Autodesk Inventor part; units mm, degrees
(part 2 of 3)
sketch "Sketch41" plane through (0, 15, 0) normal (0, 1, 0) x (1, 0, 0)
  line L0 (-15.5, 102.8) -> (-15.5, 122.8) projected
  line L1 (-15.5, 112.8) -> (-5.5, 112.8)
  line L2 (-5.5, 102.8) -> (-5.5, 122.8) projected
  line L3 (-5.5, 72.8) -> (-5.5, 92.8) projected
  line L4 (-5.5, 82.8) -> (-15.5, 82.8)
  line L5 (-15.5, 72.8) -> (-15.5, 92.8) projected
  line L6 (-35.5, 72.8) -> (-35.5, 92.8) projected
  line L7 (-35.5, 82.8) -> (-45.5, 82.8)
  line L8 (-45.5, 72.8) -> (-45.5, 92.8) projected
  line L9 (-65.5, 72.8) -> (-65.5, 92.8) projected
  line L10 (-65.5, 82.8) -> (-75.5, 82.8)
  line L11 (-75.5, 72.8) -> (-75.5, 92.8) projected
  line L12 (-75.5, 62.8) -> (-75.5, 42.8) projected
  line L13 (-75.5, 52.8) -> (-65.5, 52.8)
  line L14 (-65.5, 42.8) -> (-65.5, 62.8) projected
  line L15 (-45.5, 42.8) -> (-45.5, 62.8) projected
  line L16 (-45.5, 52.8) -> (-35.5, 52.8)
  line L17 (-35.5, 42.8) -> (-35.5, 62.8) projected
  line L18 (-15.5, 52.8) -> (-5.5, 52.8)
  line L19 (-5.5, 42.8) -> (-5.5, 62.8) projected
  line L20 (-5.5, 32.8) -> (-5.5, 12.8) projected
  line L21 (-5.5, 22.8) -> (-15.5, 22.8)
  line L22 (-15.5, 32.8) -> (-15.5, 12.8) projected
  line L23 (-45.5, 22.8) -> (-35.5, 22.8)
  line L24 (-35.5, 32.8) -> (-35.5, 12.8) projected
  line L25 (-65.5, 22.8) -> (-75.5, 22.8)
  line L26 (-75.5, 32.8) -> (-75.5, 12.8) projected
  line L27 (-70.5, 82.8) -> (-70.5, 93.8)
  line L28 (-70.5, 82.8) -> (-59.5, 82.8) construction
  line L29 (-70.5, 93.8) -> (-70.5, 71.8)
  line L30 (-40.5, 82.8) -> (-40.5, 93.8)
  line L31 (-40.5, 93.8) -> (-40.5, 71.8)
  line L32 (-10.5, 82.8) -> (-10.5, 93.8)
  line L33 (-10.5, 93.8) -> (-10.5, 71.8)
  line L34 (-10.5, 52.8) -> (-10.5, 63.8)
  line L35 (-10.5, 63.8) -> (-10.5, 41.8)
  line L36 (-40.5, 52.8) -> (-40.5, 63.8)
  line L37 (-40.5, 63.8) -> (-40.5, 41.8)
  line L38 (-70.5, 52.8) -> (-70.5, 63.8)
  line L39 (-70.5, 63.8) -> (-70.5, 41.8)
  line L40 (-70.5, 22.8) -> (-70.5, 33.8)
  line L41 (-70.5, 33.8) -> (-70.5, 11.8)
  line L42 (-40.5, 22.8) -> (-40.5, 33.8)
  line L43 (-45.5, 32.8) -> (-35.5, 32.8) projected
  line L44 (-40.5, 22.8) -> (-29.5, 22.8) construction
  line L45 (-40.5, 33.8) -> (-40.5, 11.8)
  line L46 (-10.5, 22.8) -> (-10.5, 33.8)
  line L47 (-10.5, 33.8) -> (-10.5, 11.8)
  line L48 (-10.5, 112.8) -> (-10.5, 123.8)
  line L49 (-10.5, 123.8) -> (-10.5, 101.8)
  line L50 (-10.5, 101.8) -> (0.5, 112.8)
  line L51 (0.5, 112.8) -> (-10.5, 123.8)
  line L52 (-21.5, 112.8) -> (-10.5, 101.8)
  line L53 (-10.5, 123.8) -> (-21.5, 112.8)
  line L54 (-70.5, 93.8) -> (-59.5, 82.8)
  line L55 (-70.5, 71.8) -> (-59.5, 82.8)
  line L56 (-70.5, 71.8) -> (-81.5, 82.8)
  line L57 (-81.5, 82.8) -> (-70.5, 93.8)
  line L58 (-40.5, 93.8) -> (-29.5, 82.8)
  line L59 (-29.5, 82.8) -> (-40.5, 71.8)
  line L60 (-51.5, 82.8) -> (-40.5, 71.8)
  line L61 (-51.5, 82.8) -> (-40.5, 93.8)
  line L62 (-10.5, 93.8) -> (0.5, 82.8)
  line L63 (0.5, 82.8) -> (-10.5, 71.8)
  line L64 (-21.5, 82.8) -> (-10.5, 93.8)
  line L65 (-21.5, 82.8) -> (-10.5, 71.8)
  line L66 (-10.5, 63.8) -> (0.5, 52.8)
  line L67 (-10.5, 63.8) -> (5.0563, 63.8) construction
  line L68 (0.5, 52.8) -> (-10.5, 41.8)
  line L69 (-10.5, 41.8) -> (-21.5, 52.8)
  line L70 (-21.5, 52.8) -> (-10.5, 63.8)
  line L71 (-40.5, 63.8) -> (-29.5, 52.8)
  line L72 (-29.5, 52.8) -> (-40.5, 41.8)
  line L73 (-51.5, 52.8) -> (-40.5, 63.8)
  line L74 (-51.5, 52.8) -> (-40.5, 41.8)
  line L75 (-70.5, 63.8) -> (-59.5, 52.8)
  line L76 (-59.5, 52.8) -> (-70.5, 41.8)
  line L77 (-81.5, 52.8) -> (-70.5, 41.8)
  line L78 (-81.5, 52.8) -> (-70.5, 63.8)
  line L79 (-70.5, 33.8) -> (-59.5, 22.8)
  line L80 (-59.5, 22.8) -> (-70.5, 11.8)
  line L81 (-81.5, 22.8) -> (-70.5, 11.8)
  line L82 (-81.5, 22.8) -> (-70.5, 33.8)
  line L83 (-40.5, 33.8) -> (-29.5, 22.8)
  line L84 (-40.5, 11.8) -> (-29.5, 22.8)
  line L85 (-40.5, 11.8) -> (-51.5, 22.8)
  line L86 (-51.5, 22.8) -> (-40.5, 33.8)
  line L87 (-10.5, 33.8) -> (0.5, 22.8)
  line L88 (0.5, 22.8) -> (-10.5, 11.8)
  line L89 (-21.5, 22.8) -> (-10.5, 11.8)
  line L90 (-21.5, 22.8) -> (-10.5, 33.8)
  line L91 (-5.5, 102.8) -> (-15.5, 102.8) projected
  line L92 (-15.5, 122.8) -> (-5.5, 122.8)
  line L93 (-5.5, 122.8) -> (-5.5, 102.8)
  line L94 (-5.5, 102.8) -> (-15.5, 102.8)
  line L95 (-15.5, 102.8) -> (-15.5, 122.8)
  line L96 (-15.5, 92.8) -> (-5.5, 92.8) projected
  line L97 (-15.5, 92.8) -> (-5, 92.8)
  line L98 (-5, 92.8) -> (-5, 72.8)
  line L99 (-5, 72.8) -> (-15.5, 72.8)
  line L100 (-15.5, 72.8) -> (-15.5, 92.8)
  line L101 (-45.5, 92.8) -> (-35.5, 92.8)
  line L102 (-35.5, 92.8) -> (-35.5, 72.8)
  line L103 (-35.5, 72.8) -> (-45.5, 72.8)
  line L104 (-45.5, 72.8) -> (-45.5, 92.8)
  line L105 (-75.5, 92.8) -> (-65, 92.8)
  line L106 (-65, 92.8) -> (-65, 72.8)
  line L107 (-65, 72.8) -> (-75.5, 72.8)
  line L108 (-75.5, 72.8) -> (-75.5, 92.8)
  line L109 (-75.5, 62.8) -> (-65.5, 62.8) projected
  line L110 (-75.5, 62.8) -> (-65.5, 62.8)
  line L111 (-65.5, 62.8) -> (-65.5, 42.8)
  line L112 (-65.5, 42.8) -> (-75.5, 42.8)
  line L113 (-75.5, 42.8) -> (-75.5, 62.8)
  line L114 (-45.5, 62.8) -> (-35.5, 62.8) projected
  line L115 (-45.5, 62.8) -> (-35.5, 62.8)
  line L116 (-35.5, 62.8) -> (-35.5, 42.8)
  line L117 (-35.5, 42.8) -> (-45.5, 42.8)
  line L118 (-45.5, 42.8) -> (-45.5, 62.8)
  line L119 (-15.5, 62.8) -> (-5.5, 62.8) projected
  line L120 (-5.5, 42.8) -> (-15.5, 42.8) projected
  line L121 (-15.5, 62.8) -> (-5.5, 62.8)
  line L122 (-5.5, 62.8) -> (-5.5, 42.8)
  line L123 (-5.5, 42.8) -> (-15.5, 42.8)
  line L124 (-15.5, 42.8) -> (-15.5, 62.8)
  line L125 (-15.5, 32.8) -> (-5.5, 32.8)
  line L126 (-5.5, 32.8) -> (-5.5, 12.8)
  line L127 (-5.5, 12.8) -> (-15.5, 12.8)
  line L128 (-15.5, 12.8) -> (-15.5, 32.8)
  line L129 (-45.5, 32.8) -> (-45.5, 12.8) projected
  line L130 (-45.5, 32.8) -> (-35.5, 32.8)
  line L131 (-35.5, 32.8) -> (-35.5, 12.8)
  line L132 (-35.5, 12.8) -> (-45.5, 12.8)
  line L133 (-45.5, 12.8) -> (-45.5, 32.8)
  line L134 (-75.5, 32.8) -> (-65.5, 32.8)
  line L135 (-65.5, 32.8) -> (-65.5, 12.8)
  line L136 (-65.5, 12.8) -> (-75.5, 12.8)
  line L137 (-75.5, 12.8) -> (-75.5, 32.8)
  point P0 (0, 0)
  point P1 (-41.5, 42.8)
  point P2 (-45.5, 46.8)
  point P3 (-39.5, 42.8)
  point P4 (-35.5, 46.8)
  point P5 (-39.5, 62.8)
  point P6 (-35.5, 58.8)
  point P7 (-41.5, 62.8)
  point P8 (-45.5, 58.8)
  point P9 (-41.5, 12.8)
  point P10 (-45.5, 16.8)
  point P11 (-39.5, 12.8)
  point P12 (-35.5, 16.8)
  point P13 (-39.5, 32.8)
  point P14 (-35.5, 28.8)
  point P15 (-45.5, 28.8)
  point P16 (-41.5, 32.8)
  point P17 (-71.5, 12.8)
  point P18 (-75.5, 16.8)
  point P19 (-69.5, 12.8)
  point P20 (-65.5, 16.8)
  point P21 (-65.5, 28.8)
  point P22 (-69.5, 32.8)
  point P23 (-71.5, 32.8)
  point P24 (-75.5, 28.8)
  point P25 (-71.5, 42.8)
  point P26 (-75.5, 46.8)
  point P27 (-69.5, 42.8)
  point P28 (-65.5, 46.8)
  point P29 (-69.5, 62.8)
  point P30 (-65.5, 58.8)
  point P31 (-71.5, 62.8)
  point P32 (-75.5, 58.8)
  point P33 (-71.5, 72.8)
  point P34 (-75.5, 76.8)
  point P35 (-69.5, 72.8)
  point P36 (-65.5, 76.8)
  point P37 (-71.5, 92.8)
  point P38 (-75.5, 88.8)
  point P39 (-69.5, 92.8)
  point P40 (-65.5, 88.8)
  point P41 (-39.5, 72.8)
  point P42 (-35.5, 76.8)
  point P43 (-41.5, 72.8)
  point P44 (-45.5, 76.8)
  point P45 (-39.5, 92.8)
  point P46 (-35.5, 88.8)
  point P47 (-41.5, 92.8)
  point P48 (-45.5, 88.8)
  point P49 (-11.5, 12.8)
  point P50 (-15.5, 16.8)
  point P51 (-9.5, 12.8)
  point P52 (-5.5, 16.8)
  point P53 (-9.5, 32.8)
  point P54 (-5.5, 28.8)
  point P55 (-11.5, 32.8)
  point P56 (-15.5, 28.8)
  point P57 (-9.5, 62.8)
  point P58 (-5.5, 58.8)
  point P59 (-15.5, 58.8)
  point P60 (-11.5, 62.8)
  point P61 (-15.5, 46.8)
  point P62 (-11.5, 42.8)
  point P63 (-9.5, 42.8)
  point P64 (-5.5, 46.8)
  point P65 (-9.5, 72.8)
  point P66 (-5.5, 76.8)
  point P67 (-9.5, 92.8)
  point P68 (-5.5, 88.8)
  point P69 (-11.5, 92.8)
  point P70 (-15.5, 88.8)
  point P71 (-11.5, 72.8)
  point P72 (-15.5, 76.8)
  point P73 (-11.5, 102.8)
  point P74 (-15.5, 106.8)
  point P75 (-9.5, 102.8)
  point P76 (-5.5, 106.8)
  point P77 (-9.5, 122.8)
  point P78 (-5.5, 118.8)
  point P79 (-11.5, 122.8)
  point P80 (-15.5, 118.8)
  dimension "d189" = 11
  dimension "d190" = 90
  dimension "d191" = 22
  dimension "d192" = 11
  dimension "d193" = 22
  dimension "d194" = 11
  dimension "d195" = 22
  dimension "d196" = 11
  dimension "d197" = 22
  dimension "d198" = 11
  dimension "d199" = 22
  dimension "d200" = 11
  dimension "d201" = 22
  dimension "d202" = 11
  dimension "d203" = 22
  dimension "d204" = 11
  dimension "d205" = 90
  dimension "d206" = 22
  dimension "d207" = 11
  dimension "d208" = 22
  dimension "d209" = 11
  dimension "d210" = 22
  dimension "d211" = 45
  dimension "d212" = 45
  constraints: 226 end point, 36 perpendicular, 27 midpoint, 23 point on line, 22 parallel, 13 horizontal, 9 vertical, 3 equal length
  measures "d189" distance of L27.start L27.end
  measures "d190" angle of L28 L27
  measures "d191" distance of L27.end L29.end
  measures "d192" distance of L30.start L30.end
  measures "d193" distance of L30.end L31.end
  measures "d194" distance of L32.start L32.end
  measures "d195" distance of L32.end L33.end
  measures "d196" distance of L34.start L34.end
  measures "d197" distance of L34.end L35.end
  measures "d198" distance of L36.start L36.end
  measures "d199" distance of L36.end L37.end
  measures "d200" distance of L38.start L38.end
  measures "d201" distance of L38.end L39.end
  measures "d202" distance of L40.start L40.end
  measures "d203" distance of L40.end L41.end
  measures "d204" distance of L42.start L42.end
  measures "d205" angle of L44 L42
  measures "d206" distance of L42.end L45.end
  measures "d207" distance of L46.start L46.end
  measures "d208" distance of L46.end L47.end
  measures "d209" distance of L48.start L48.end
  measures "d210" distance of L48.end L49.end
  measures "d211" angle of L50 L49
  measures "d212" angle of L66 L67
extrude "Extrusion39" add sketch "Sketch41" along normal blind 3 contours L0 L52 L91 | L0 L92 L53 | L50 L2 L91 | L51 L92 L2 | L99 L63 L3 | L62 L96 L3 | L99 L5 L65 | L5 L96 L64 | L103 L59 L6 | L58 L101 L6 | L103 L8 L60 | L8 L101 L61 | L107 L55 L9 | L54 L105 L9 | L107 L11 L56 | L11 L105 L57 | L109 L78 L12 | L77 L112 L12 | L109 L14 L75 | L14 L112 L76 | L15 L74 L117 | L15 L114 L73 | L72 L17 L117 | L71 L114 L17 | L69 L120 L124 | L124 L119 L70 | L19 L120 L68 | L66 L119 L19 | L20 L87 L125 | L20 L127 L88 | L90 L22 L125 | L89 L127 L22 | L129 L43 L86 | L85 L132 L129 | L83 L43 L24 | L24 L132 L84 | L79 L134 L135 | L135 L136 L80 | L26 L134 L82 | L81 L136 L26
chamfer "Chamfer9" distance 2.5 distance2 3 1 edges at (-73.5, 18, -90.8) measured on face at (-73.8536, 18, -91.1536)
chamfer "Chamfer10" distance 2.5 distance2 3 1 edges at (-67.5, 18, -90.8) measured on face at (-67.1464, 18, -91.1536)
chamfer "Chamfer11" distance 2.5 distance2 3 1 edges at (-67.5, 18, -74.8) measured on face at (-67.1464, 18, -74.4464)
chamfer "Chamfer12" distance 2.5 distance2 3 1 edges at (-73.5, 18, -74.8) measured on face at (-73.8536, 18, -74.4464)
chamfer "Chamfer13" distance 2.5 distance2 3 1 edges at (-73.5, 18, -60.8) measured on face at (-73.8536, 18, -61.1536)
chamfer "Chamfer14" distance 2.5 distance2 3 1 edges at (-67.5, 18, -60.8) measured on face at (-67.1464, 18, -61.1536)
chamfer "Chamfer15" distance 2.5 distance2 3 1 edges at (-67.5, 18, -44.8) measured on face at (-67.1464, 18, -44.4464)
chamfer "Chamfer16" distance 2.5 distance2 3 1 edges at (-73.5, 18, -44.8) measured on face at (-73.8536, 18, -44.4464)
chamfer "Chamfer17" distance 2.5 distance2 3 1 edges at (-73.5, 18, -30.8) measured on face at (-73.8536, 18, -31.1536)
chamfer "Chamfer18" distance 2.5 distance2 3 1 edges at (-67.5, 18, -30.8) measured on face at (-67.1464, 18, -31.1536)
chamfer "Chamfer19" distance 2.5 distance2 3 1 edges at (-67.5, 18, -14.8) measured on face at (-67.1464, 18, -14.4464)
chamfer "Chamfer20" distance 2.5 distance2 3 1 edges at (-73.5, 18, -14.8) measured on face at (-73.8536, 18, -14.4464)
chamfer "Chamfer21" distance 2.5 distance2 3 1 edges at (-43.5, 18, -30.8) measured on face at (-43.8536, 18, -31.1536)
chamfer "Chamfer22" distance 2.5 distance2 3 1 edges at (-43.5, 18, -14.8) measured on face at (-43.8536, 18, -14.4464)
chamfer "Chamfer23" distance 2.5 distance2 3 1 edges at (-37.5, 18, -14.8) measured on face at (-37.1464, 18, -14.4464)
chamfer "Chamfer24" distance 2.5 distance2 3 1 edges at (-37.5, 18, -30.8) measured on face at (-37.1464, 18, -31.1536)
chamfer "Chamfer25" distance 2.5 distance2 3 1 edges at (-43.5, 18, -60.8) measured on face at (-43.8536, 18, -61.1536)
chamfer "Chamfer26" distance 2.5 distance2 3 1 edges at (-43.5, 18, -44.8) measured on face at (-43.8536, 18, -44.4464)
chamfer "Chamfer27" distance 2.5 distance2 3 1 edges at (-37.5, 18, -44.8) measured on face at (-37.1464, 18, -44.4464)
chamfer "Chamfer28" distance 2.5 distance2 3 1 edges at (-37.5, 18, -60.8) measured on face at (-37.1464, 18, -61.1536)
chamfer "Chamfer29" distance 2.5 distance2 3 1 edges at (-13.5, 18, -30.8) measured on face at (-13.8536, 18, -31.1536)
chamfer "Chamfer30" distance 2.5 distance2 3 1 edges at (-13.5, 18, -14.8) measured on face at (-13.8536, 18, -14.4464)
chamfer "Chamfer31" distance 2.5 distance2 3 1 edges at (-7.5, 18, -14.8) measured on face at (-7.1464, 18, -14.4464)
chamfer "Chamfer32" distance 2.5 distance2 3 1 edges at (-7.5, 18, -30.8) measured on face at (-7.1464, 18, -31.1536)
chamfer "Chamfer33" distance 2.5 distance2 3 1 edges at (-13.5, 18, -60.8) measured on face at (-13.8536, 18, -61.1536)
chamfer "Chamfer34" distance 2.5 distance2 3 1 edges at (-13.5, 18, -44.8) measured on face at (-13.8536, 18, -44.4464)
chamfer "Chamfer35" distance 2.5 distance2 3 1 edges at (-7.5, 18, -44.8) measured on face at (-7.1464, 18, -44.4464)
chamfer "Chamfer36" distance 2.5 distance2 3 1 edges at (-7.5, 18, -60.8) measured on face at (-7.1464, 18, -61.1536)
chamfer "Chamfer37" distance 2.5 distance2 3 1 edges at (-13.5, 18, -90.8) measured on face at (-13.8536, 18, -91.1536)
chamfer "Chamfer38" distance 2.5 distance2 3 1 edges at (-13.5, 18, -74.8) measured on face at (-13.8536, 18, -74.4464)
chamfer "Chamfer39" distance 2.5 distance2 3 1 edges at (-7.5, 18, -74.8) measured on face at (-7.1464, 18, -74.4464)
chamfer "Chamfer40" distance 2.5 distance2 3 1 edges at (-7.5, 18, -90.8) measured on face at (-7.1464, 18, -91.1536)
chamfer "Chamfer41" distance 2.5 distance2 3 1 edges at (-13.5, 18, -120.8) measured on face at (-13.8536, 18, -121.1536)
chamfer "Chamfer42" distance 2.5 distance2 3 1 edges at (-7.5, 18, -120.8) measured on face at (-7.1464, 18, -121.1536)
chamfer "Chamfer43" distance 2.5 distance2 3 1 edges at (-7.5, 18, -104.8) measured on face at (-7.1464, 18, -104.4464)
chamfer "Chamfer44" distance 2.5 distance2 3 1 edges at (-13.5, 18, -104.8) measured on face at (-13.8536, 18, -104.4464)
chamfer "Chamfer45" distance 2.5 distance2 3 1 edges at (-43.5, 18, -90.8) measured on face at (-43.8536, 18, -91.1536)
chamfer "Chamfer46" distance 2.5 distance2 3 1 edges at (-43.5, 18, -74.8) measured on face at (-43.8536, 18, -74.4464)
chamfer "Chamfer47" distance 2.5 distance2 3 1 edges at (-37.5, 18, -90.8) measured on face at (-37.1464, 18, -91.1536)
chamfer "Chamfer48" distance 2.5 distance2 3 1 edges at (-37.5, 18, -74.8) measured on face at (-37.1464, 18, -74.4464)
sketch "Sketch42" plane through (0, 15, 0) normal (0, 1, 0) x (1, 0, 0)
  line L0 (-69.5, 102.8) -> (-65.5, 106.8) projected
  line L1 (-65.5, 106.8) -> (-65.5, 118.8) projected
  line L2 (-65.5, 118.8) -> (-69.5, 122.8) projected
  line L3 (-71.5, 122.8) -> (-69.5, 122.8) projected
  line L4 (-71.5, 122.8) -> (-75.5, 118.8) projected
  line L5 (-75.5, 118.8) -> (-75.5, 106.8) projected
  line L6 (-75.5, 106.8) -> (-71.5, 102.8) projected
  line L7 (-69.5, 102.8) -> (-71.5, 102.8) projected
  line L8 (-39.5, 102.8) -> (-35.5, 106.8) projected
  line L9 (-35.5, 106.8) -> (-35.5, 118.8) projected
  line L10 (-35.5, 118.8) -> (-39.5, 122.8) projected
  line L11 (-41.5, 122.8) -> (-39.5, 122.8) projected
  line L12 (-41.5, 122.8) -> (-45.5, 118.8) projected
  line L13 (-45.5, 118.8) -> (-45.5, 106.8) projected
  line L14 (-45.5, 106.8) -> (-41.5, 102.8) projected
  line L15 (-39.5, 102.8) -> (-41.5, 102.8) projected
  line L16 (-9.5, 102.8) -> (-5.5, 106.8) projected
  line L17 (-5.5, 106.8) -> (-5.5, 118.8) projected
  line L18 (-5.5, 118.8) -> (-9.5, 122.8) projected
  line L19 (-11.5, 122.8) -> (-9.5, 122.8) projected
  line L20 (-11.5, 122.8) -> (-15.5, 118.8) projected
  line L21 (-15.5, 118.8) -> (-15.5, 106.8) projected
  line L22 (-15.5, 106.8) -> (-11.5, 102.8) projected
  line L23 (-9.5, 102.8) -> (-11.5, 102.8) projected
  line L24 (-5.5, 88.8) -> (-9.5, 92.8) projected
  line L25 (-11.5, 92.8) -> (-9.5, 92.8) projected
  line L26 (-11.5, 92.8) -> (-15.5, 88.8) projected
  line L27 (-15.5, 88.8) -> (-15.5, 76.8) projected
  line L28 (-15.5, 76.8) -> (-11.5, 72.8) projected
  line L29 (-9.5, 72.8) -> (-11.5, 72.8) projected
  line L30 (-9.5, 72.8) -> (-5.5, 76.8) projected
  line L31 (-5.5, 76.8) -> (-5.5, 88.8) projected
  line L32 (-45.5, 76.8) -> (-41.5, 72.8) projected
  line L33 (-39.5, 72.8) -> (-41.5, 72.8) projected
  line L34 (-39.5, 72.8) -> (-35.5, 76.8) projected
  line L35 (-35.5, 76.8) -> (-35.5, 88.8) projected
  line L36 (-35.5, 88.8) -> (-39.5, 92.8) projected
  line L37 (-41.5, 92.8) -> (-39.5, 92.8) projected
  line L38 (-41.5, 92.8) -> (-45.5, 88.8) projected
  line L39 (-45.5, 88.8) -> (-45.5, 76.8) projected
  line L40 (-69.5, 72.8) -> (-65.5, 76.8) projected
  line L41 (-65.5, 76.8) -> (-65.5, 88.8) projected
  line L42 (-65.5, 88.8) -> (-69.5, 92.8) projected
  line L43 (-71.5, 92.8) -> (-69.5, 92.8) projected
  line L44 (-71.5, 92.8) -> (-75.5, 88.8) projected
  line L45 (-75.5, 88.8) -> (-75.5, 76.8) projected
  line L46 (-75.5, 76.8) -> (-71.5, 72.8) projected
  line L47 (-69.5, 72.8) -> (-71.5, 72.8) projected
  line L48 (-75.5, 58.8) -> (-75.5, 46.8) projected
  line L49 (-69.5, 42.8) -> (-65.5, 46.8) projected
  line L50 (-65.5, 46.8) -> (-65.5, 58.8) projected
  line L51 (-65.5, 58.8) -> (-69.5, 62.8) projected
  line L52 (-71.5, 62.8) -> (-69.5, 62.8) projected
  line L53 (-71.5, 62.8) -> (-75.5, 58.8) projected
  line L54 (-75.5, 58.8) -> (-75.5, 46.8) projected
  line L55 (-75.5, 46.8) -> (-71.5, 42.8) projected
  line L56 (-69.5, 42.8) -> (-71.5, 42.8) projected
  line L57 (-39.5, 42.8) -> (-35.5, 46.8) projected
  line L58 (-35.5, 46.8) -> (-35.5, 58.8) projected
  line L59 (-35.5, 58.8) -> (-39.5, 62.8) projected
  line L60 (-41.5, 62.8) -> (-39.5, 62.8) projected
  line L61 (-41.5, 62.8) -> (-45.5, 58.8) projected
  line L62 (-45.5, 58.8) -> (-45.5, 46.8) projected
  line L63 (-45.5, 46.8) -> (-41.5, 42.8) projected
  line L64 (-39.5, 42.8) -> (-41.5, 42.8) projected
  line L65 (-11.5, 62.8) -> (-15.5, 58.8) projected
  line L66 (-15.5, 58.8) -> (-15.5, 46.8) projected
  line L67 (-15.5, 46.8) -> (-11.5, 42.8) projected
  line L68 (-9.5, 42.8) -> (-11.5, 42.8) projected
  line L69 (-9.5, 42.8) -> (-5.5, 46.8) projected
  line L70 (-5.5, 46.8) -> (-5.5, 58.8) projected
  line L71 (-5.5, 58.8) -> (-9.5, 62.8) projected
  line L72 (-11.5, 62.8) -> (-9.5, 62.8) projected
  line L73 (-9.5, 12.8) -> (-5.5, 16.8) projected
  line L74 (-5.5, 16.8) -> (-5.5, 28.8) projected
  line L75 (-5.5, 28.8) -> (-9.5, 32.8) projected
  line L76 (-11.5, 32.8) -> (-9.5, 32.8) projected
  line L77 (-11.5, 32.8) -> (-15.5, 28.8) projected
  line L78 (-15.5, 28.8) -> (-15.5, 16.8) projected
  line L79 (-15.5, 16.8) -> (-11.5, 12.8) projected
  line L80 (-9.5, 12.8) -> (-11.5, 12.8) projected
  line L81 (-39.5, 12.8) -> (-35.5, 16.8) projected
  line L82 (-35.5, 16.8) -> (-35.5, 28.8) projected
  line L83 (-35.5, 28.8) -> (-39.5, 32.8) projected
  line L84 (-41.5, 32.8) -> (-39.5, 32.8) projected
  line L85 (-41.5, 32.8) -> (-45.5, 28.8) projected
  line L86 (-45.5, 28.8) -> (-45.5, 16.8) projected
  line L87 (-45.5, 16.8) -> (-41.5, 12.8) projected
  line L88 (-39.5, 12.8) -> (-41.5, 12.8) projected
  line L89 (-69.5, 12.8) -> (-65.5, 16.8) projected
  line L90 (-65.5, 16.8) -> (-65.5, 28.8) projected
  line L91 (-65.5, 28.8) -> (-69.5, 32.8) projected
  line L92 (-71.5, 32.8) -> (-69.5, 32.8) projected
  line L93 (-71.5, 32.8) -> (-75.5, 28.8) projected
  line L94 (-75.5, 28.8) -> (-75.5, 16.8) projected
  line L95 (-75.5, 16.8) -> (-71.5, 12.8) projected
  line L96 (-69.5, 12.8) -> (-71.5, 12.8) projected
  point P0 (0, 0)
extrude "Extrusion40" cut sketch "Sketch42" against normal blind 3
sketch "Sketch43" plane through (0, 12, 0) normal (0, 1, 0) x (1, 0, 0)
  line L0 (-91.1439, 136.9955) -> (37.6505, 136.9955)
  line L1 (37.6505, 136.9955) -> (37.6505, 0)
  line L2 (37.6505, 0) -> (-91.1439, 0)
  line L3 (-91.1439, 0) -> (-91.1439, 136.9955)
  point P0 (0, 0)
  constraints: 8 end point, 2 parallel, 1 horizontal, 1 perpendicular
extrude "Extrusion41" cut sketch "Sketch43" along normal blind 10
sketch "Sketch44" plane through (0, 12, 0) normal (0, 1, 0) x (1, 0, 0)
  line L0 (-75.5, 102.8) -> (-75.5, 122.8) projected
  line L1 (-65.5, 12.8) -> (-75.5, 12.8) projected
  line L2 (-75.5, 122.8) -> (-74.5, 122.8)
  line L3 (-74.5, 122.8) -> (-74.5, 12.8)
  line L4 (-74.5, 12.8) -> (-75.5, 12.8)
  line L5 (-75.5, 12.8) -> (-75.5, 122.8)
  line L6 (-65.5, 122.8) -> (-65.5, 102.8) projected
  line L7 (-65.5, 122.8) -> (-66.5, 122.8)
  line L8 (-66.5, 122.8) -> (-66.5, 12.8)
  line L9 (-66.5, 12.8) -> (-65.5, 12.8)
  line L10 (-65.5, 12.8) -> (-65.5, 122.8)
  line L11 (-35.5, 12.8) -> (-45.5, 12.8) projected
  line L12 (-45.5, 12.8) -> (-44.5, 12.8)
  line L13 (-44.5, 12.8) -> (-44.5, 122.8)
  line L14 (-44.5, 122.8) -> (-45.5, 122.8)
  line L15 (-45.5, 122.8) -> (-45.5, 12.8)
  line L16 (-35.5, 122.8) -> (-36.5, 122.8)
  line L17 (-36.5, 122.8) -> (-36.5, 12.8)
  line L18 (-36.5, 12.8) -> (-35.5, 12.8)
  line L19 (-35.5, 12.8) -> (-35.5, 122.8)
  line L20 (-15.5, 122.8) -> (-5.5, 122.8) projected
  line L21 (-5.5, 12.8) -> (-15.5, 12.8) projected
  line L22 (-15.5, 122.8) -> (-14.5, 122.8)
  line L23 (-14.5, 122.8) -> (-14.5, 12.8)
  line L24 (-14.5, 12.8) -> (-15.5, 12.8)
  line L25 (-15.5, 12.8) -> (-15.5, 122.8)
  line L26 (-5.5, 122.8) -> (-6.5, 122.8)
  line L27 (-6.5, 122.8) -> (-6.5, 12.8)
  line L28 (-6.5, 12.8) -> (-5.5, 12.8)
  line L29 (-5.5, 12.8) -> (-5.5, 122.8)
  point P0 (0, 0)
  dimension "d339" = 1
  dimension "d340" = 1
  dimension "d341" = 1
  dimension "d342" = 1
  dimension "d343" = 1
  dimension "d344" = 1
  constraints: 48 end point, 12 parallel, 7 point on line, 6 horizontal, 6 perpendicular
  measures "d339" distance of L3.end L4.end
  measures "d340" distance of L9.end L8.end
  measures "d341" distance of L14.end L13.end
  measures "d342" distance of L18.end L17.end
  measures "d343" distance of L23.end L24.end
  measures "d344" distance of L28.end L27.end
extrude "Extrusion42" cut sketch "Sketch44" against normal blind 7 contours L0 L2 L3 L1 L5 | L1 L8 L7 L6 L10 | L11 L17 L16 L19 | L11 L15 L14 L13 | L20 L23 L21 L25 | L20 L29 L21 L27
sketch "Sketch45" plane through (0, 12, 0) normal (0, 1, 0) x (1, 0, 0)
  line L0 (-74.5, 122.8) -> (-74.5, 102.8) projected
  line L1 (-74.5, 122.8) -> (-66.5, 122.8)
  line L2 (-66.5, 122.8) -> (-66.5, 125.8)
  line L3 (-66.5, 125.8) -> (-74.5, 125.8)
  line L4 (-74.5, 125.8) -> (-74.5, 122.8)
  line L5 (-66.5, 102.8) -> (-66.5, 122.8) projected
  line L6 (-66.5, 102.8) -> (-74.5, 102.8)
  line L7 (-74.5, 102.8) -> (-74.5, 99.8)
  line L8 (-74.5, 99.8) -> (-66.5, 99.8)
  line L9 (-66.5, 99.8) -> (-66.5, 102.8)
  line L10 (-74.5, 92.8) -> (-66.5, 92.8) projected
  line L11 (-74.5, 92.8) -> (-66.5, 92.8)
  line L12 (-66.5, 92.8) -> (-66.5, 95.8)
  line L13 (-66.5, 95.8) -> (-74.5, 95.8)
  line L14 (-74.5, 95.8) -> (-74.5, 92.8)
  line L15 (-66.5, 72.8) -> (-74.5, 72.8) projected
  line L16 (-74.5, 72.8) -> (-66.5, 72.8)
  line L17 (-66.5, 72.8) -> (-66.5, 69.8)
  line L18 (-66.5, 69.8) -> (-74.5, 69.8)
  line L19 (-74.5, 69.8) -> (-74.5, 72.8)
  line L20 (-74.5, 62.8) -> (-66.5, 62.8)
  line L21 (-66.5, 62.8) -> (-66.5, 65.8)
  line L22 (-66.5, 65.8) -> (-74.5, 65.8)
  line L23 (-74.5, 65.8) -> (-74.5, 62.8)
  line L24 (-66.5, 42.8) -> (-74.5, 42.8) projected
  line L25 (-74.5, 42.8) -> (-66.5, 42.8)
  line L26 (-66.5, 42.8) -> (-66.5, 39.8)
  line L27 (-66.5, 39.8) -> (-74.5, 39.8)
  line L28 (-74.5, 39.8) -> (-74.5, 42.8)
  line L29 (-74.5, 32.8) -> (-66.5, 32.8) projected
  line L30 (-74.5, 32.8) -> (-66.5, 32.8)
  line L31 (-66.5, 32.8) -> (-66.5, 35.8)
  line L32 (-66.5, 35.8) -> (-74.5, 35.8)
  line L33 (-74.5, 35.8) -> (-74.5, 32.8)
  line L34 (-66.5, 12.8) -> (-74.5, 12.8) projected
  line L35 (-74.5, 12.8) -> (-66.5, 12.8)
  line L36 (-66.5, 12.8) -> (-66.5, 9.8)
  line L37 (-66.5, 9.8) -> (-74.5, 9.8)
  line L38 (-74.5, 9.8) -> (-74.5, 12.8)
  point P0 (0, 0)
  dimension "d347" = 3
  dimension "d348" = 3
  dimension "d349" = 8
  dimension "d350" = 3
  dimension "d351" = 3
  dimension "d352" = 8
  dimension "d353" = 3
  dimension "d354" = 8
  dimension "d355" = 3
  dimension "d356" = 8
  dimension "d357" = 3
  dimension "d358" = 8
  dimension "d359" = 3
  constraints: 64 end point, 16 parallel, 8 horizontal, 8 perpendicular, 2 point on line
  measures "d347" distance of L2.end L1.end
  measures "d348" distance of L7.end L6.end
  measures "d349" distance of L13.end L12.end
  measures "d350" distance of L12.end L11.end
  measures "d351" distance of L16.end L17.end
  measures "d352" distance of L22.end L21.end
  measures "d353" distance of L21.end L20.end
  measures "d354" distance of L26.end L27.end
  measures "d355" distance of L25.end L26.end
  measures "d356" distance of L32.end L31.end
  measures "d357" distance of L31.end L30.end
  measures "d358" distance of L36.end L37.end
  measures "d359" distance of L35.end L36.end
extrude "Extrusion43" add sketch "Sketch45" against normal blind 7 contours L4 L3 L2 L1 | L6 L9 L8 L7 | L14 L13 L12 L10 | L17 L18 L19 L15 | L23 L22 L21 L20 | L26 L27 L28 L24 | L33 L32 L31 L29 | L36 L37 L38 L34
sketch "Sketch46" plane through (0, 12, 0) normal (0, 1, 0) x (1, 0, 0)
  line L0 (-74.5, 99.8) -> (-74.5, 125.8) projected
  line L1 (-74.5, 112.8) -> (-66.5, 112.8)
  line L2 (-66.5, 99.8) -> (-66.5, 125.8) projected
  line L3 (-70.5, 112.8) -> (-70.5, 124.3)
  line L4 (-66.5, 125.8) -> (-74.5, 125.8) projected
  line L5 (-70.5, 124.3) -> (-74.5, 120.3)
  line L6 (-70.5, 124.3) -> (-64.8431, 124.3) construction
  line L7 (-74.5, 120.3) -> (-70.5, 124.3)
  line L8 (-70.5, 124.3) -> (-66.5, 120.3)
  line L9 (-70.5, 112.8) -> (-70.5, 101.3)
  line L10 (-74.5, 99.8) -> (-66.5, 99.8) projected
  line L11 (-70.5, 101.3) -> (-66.5, 105.3)
  line L12 (-70.5, 101.3) -> (-74.5, 105.3)
  point P0 (0, 0)
  dimension "d362" = 11.5
  dimension "d363" = 135
  dimension "d364" = 11.5
  constraints: 18 end point, 4 perpendicular, 3 midpoint, 3 point on line, 1 collinear, 1 equal length, 1 horizontal
  measures "d362" distance of L3.start L3.end
  measures "d363" angle of L5 L6
  measures "d364" distance of L3.start L9.end
extrude "Extrusion44" add sketch "Sketch46" along normal blind 4 contours L0 L12 L11 L2 L10 | L0 L4 L2 L8 L5
chamfer "Chamfer49" distance 2 distance2 3 2 edges at (-68.5, 16, -122.3) (-72.5, 16, -122.3)
chamfer "Chamfer50" distance 2 distance2 3 2 edges at (-68.5, 16, -103.3) (-72.5, 16, -103.3)
sketch "Sketch47" plane through (0, 12, 0) normal (0, 1, 0) x (1, 0, 0)
  line L0 (-66.5, 95.8) -> (-66.5, 69.8) projected
  line L1 (-66.5, 82.8) -> (-74.5, 82.8)
  line L2 (-74.5, 69.8) -> (-74.5, 95.8) projected
  line L3 (-70.5, 82.8) -> (-70.5, 94.3)
  line L4 (-70.5, 94.3) -> (-70.5, 71.3)
  line L5 (-70.5, 71.3) -> (-66.5, 75.3)
  line L6 (-66.5, 75.3) -> (-70.5, 71.3)
  line L7 (-74.5, 75.3) -> (-70.5, 71.3)
  line L8 (-70.5, 94.3) -> (-74.5, 90.3)
  line L9 (-70.5, 94.3) -> (-66.5, 90.3)
  line L10 (-74.5, 69.8) -> (-66.5, 69.8) projected
  line L11 (-74.5, 95.8) -> (-66.5, 95.8)
  line L12 (-66.5, 95.8) -> (-66.5, 69.8)
  line L13 (-66.5, 69.8) -> (-74.5, 69.8)
  line L14 (-74.5, 69.8) -> (-74.5, 95.8)
  point P0 (0, 0)
  dimension "d373" = 11.5
  dimension "d374" = 23
  dimension "d375" = 45
  constraints: 24 end point, 3 equal length, 3 midpoint, 3 perpendicular, 2 point on line, 1 horizontal, 1 vertical
  measures "d373" distance of L3.start L3.end
  measures "d374" distance of L3.end L4.end
  measures "d375" angle of L5 L4
extrude "Extrusion45" add sketch "Sketch47" along normal blind 4 contours L0 L9 L8 L2 L11 | L0 L10 L2 L7 L5
chamfer "Chamfer51" distance 2 distance2 3 2 edges at (-72.5, 16, -92.3) (-68.5, 16, -92.3)
chamfer "Chamfer52" distance 2 distance2 3 2 edges at (-68.5, 16, -73.3) (-72.5, 16, -73.3)
sketch "Sketch48" plane through (0, 12, 0) normal (0, 1, 0) x (1, 0, 0)
  line L0 (-66.5, 39.8) -> (-66.5, 65.8) projected
  line L1 (-66.5, 52.8) -> (-74.5, 52.8)
  line L2 (-74.5, 65.8) -> (-74.5, 39.8) projected
  line L3 (-70.5, 52.8) -> (-70.5, 64.3)
  line L4 (-70.5, 64.3) -> (-70.5, 52.8)
  line L5 (-70.5, 52.8) -> (-70.5, 41.3)
  line L6 (-70.5, 41.3) -> (-66.5, 45.3)
  line L7 (-66.5, 45.3) -> (-70.5, 41.3)
  line L8 (-74.5, 45.3) -> (-70.5, 41.3)
  line L9 (-70.5, 64.3) -> (-74.5, 60.3)
  line L10 (-70.5, 64.3) -> (-64.8431, 64.3) construction
  line L11 (-74.5, 60.3) -> (-70.5, 64.3)
  line L12 (-66.5, 60.3) -> (-70.5, 64.3)
  line L13 (-74.5, 65.8) -> (-66.5, 65.8)
  line L14 (-66.5, 65.8) -> (-66.5, 39.8)
  line L15 (-66.5, 39.8) -> (-74.5, 39.8)
  line L16 (-74.5, 39.8) -> (-74.5, 65.8)
  line L17 (-66.5, 9.8) -> (-66.5, 35.8) projected
  line L18 (-74.5, 35.8) -> (-66.5, 35.8)
  line L19 (-66.5, 35.8) -> (-66.5, 9.8)
  line L20 (-66.5, 9.8) -> (-74.5, 9.8)
  line L21 (-74.5, 9.8) -> (-74.5, 35.8)
  line L22 (-74.5, 35.8) -> (-74.5, 9.8) projected
  line L23 (-74.5, 22.8) -> (-66.5, 22.8)
  line L24 (-70.5, 22.8) -> (-70.5, 34.3)
  line L25 (-70.5, 34.3) -> (-70.5, 11.3)
  line L26 (-70.5, 11.3) -> (-74.5, 15.3)
  line L27 (-70.5, 11.3) -> (-66.5, 15.3)
  line L28 (-70.5, 34.3) -> (-66.5, 30.3)
  line L29 (-70.5, 34.3) -> (-74.5, 30.3)
  point P0 (0, 0)
  dimension "d384" = 11.5
  dimension "d385" = 11.5
  dimension "d386" = 45
  dimension "d387" = 135
  dimension "d388" = 11.5
  dimension "d389" = 23
  constraints: 52 end point, 8 equal length, 6 midpoint, 6 perpendicular, 6 point on line, 3 horizontal, 2 vertical
  measures "d384" distance of L3.start L3.end
  measures "d385" distance of L3.start L5.end
  measures "d386" angle of L6 L5
  measures "d387" angle of L9 L10
  measures "d388" distance of L24.start L24.end
  measures "d389" distance of L24.end L25.end
extrude "Extrusion46" add sketch "Sketch48" along normal blind 4 contours L15 L2 L8 L6 L0 | L12 L9 L2 L13 L0 | L20 L21 L26 L27 L17 | L28 L29 L21 L18 L17
chamfer "Chamfer53" distance 2 distance2 3 2 edges at (-68.5, 16, -62.3) (-72.5, 16, -62.3)
chamfer "Chamfer54" distance 2 distance2 3 2 edges at (-72.5, 16, -43.3) (-68.5, 16, -43.3)
chamfer "Chamfer55" distance 2 distance2 3 2 edges at (-72.5, 16, -32.3) (-68.5, 16, -32.3)
chamfer "Chamfer56" distance 2 distance2 3 2 edges at (-72.5, 16, -13.3) (-68.5, 16, -13.3)
sketch "Sketch49" plane through (0, 12, 0) normal (0, 1, 0) x (1, 0, 0)
  line L0 (-44.5, 122.8) -> (-44.5, 102.8) projected
  line L1 (-44.5, 122.8) -> (-36.5, 122.8)
  line L2 (-36.5, 122.8) -> (-36.5, 125.8)
  line L3 (-36.5, 125.8) -> (-44.5, 125.8)
  line L4 (-44.5, 125.8) -> (-44.5, 122.8)
  line L5 (-44.5, 102.8) -> (-36.5, 102.8)
  line L6 (-36.5, 102.8) -> (-36.5, 99.8)
  line L7 (-36.5, 99.8) -> (-44.5, 99.8)
  line L8 (-44.5, 99.8) -> (-44.5, 102.8)
  line L9 (-44.5, 92.8) -> (-36.5, 92.8) projected
  line L10 (-44.5, 92.8) -> (-36.5, 92.8)
  line L11 (-36.5, 92.8) -> (-36.5, 95.8)
  line L12 (-36.5, 95.8) -> (-44.5, 95.8)
  line L13 (-44.5, 95.8) -> (-44.5, 92.8)
  line L14 (-44.5, 92.8) -> (-44.5, 72.8) projected
  line L15 (-44.5, 72.8) -> (-36.5, 72.8)
  line L16 (-36.5, 72.8) -> (-36.5, 69.8)
  line L17 (-36.5, 69.8) -> (-44.5, 69.8)
  line L18 (-44.5, 69.8) -> (-44.5, 72.8)
  line L19 (-44.5, 62.8) -> (-36.5, 62.8) projected
  line L20 (-44.5, 62.8) -> (-36.5, 62.8)
  line L21 (-36.5, 62.8) -> (-36.5, 65.8)
  line L22 (-36.5, 65.8) -> (-44.5, 65.8)
  line L23 (-44.5, 65.8) -> (-44.5, 62.8)
  line L24 (-36.5, 42.8) -> (-44.5, 42.8) projected
  line L25 (-44.5, 42.8) -> (-36.5, 42.8)
  line L26 (-36.5, 42.8) -> (-36.5, 39.8)
  line L27 (-36.5, 39.8) -> (-44.5, 39.8)
  line L28 (-44.5, 39.8) -> (-44.5, 42.8)
  line L29 (-44.5, 32.8) -> (-36.5, 32.8)
  line L30 (-36.5, 32.8) -> (-36.5, 35.8)
  line L31 (-36.5, 35.8) -> (-44.5, 35.8)
  line L32 (-44.5, 35.8) -> (-44.5, 32.8)
  line L33 (-44.5, 32.8) -> (-44.5, 12.8) projected
  line L34 (-44.5, 12.8) -> (-36.5, 12.8)
  line L35 (-36.5, 12.8) -> (-36.5, 9.8)
  line L36 (-36.5, 9.8) -> (-44.5, 9.8)
  line L37 (-44.5, 9.8) -> (-44.5, 12.8)
  line L38 (-14.5, 122.8) -> (-14.5, 102.8) projected
  line L39 (-14.5, 122.8) -> (-6.5, 122.8)
  line L40 (-6.5, 122.8) -> (-6.5, 125.8)
  line L41 (-6.5, 125.8) -> (-14.5, 125.8)
  line L42 (-14.5, 125.8) -> (-14.5, 122.8)
  line L43 (-14.5, 92.8) -> (-14.5, 72.8) projected
  line L44 (-14.5, 92.8) -> (-6.5, 92.8)
  line L45 (-6.5, 92.8) -> (-6.5, 95.8)
  line L46 (-6.5, 95.8) -> (-14.5, 95.8)
  line L47 (-14.5, 95.8) -> (-14.5, 92.8)
  line L48 (-14.5, 72.8) -> (-6.5, 72.8)
  line L49 (-6.5, 72.8) -> (-6.5, 69.8)
  line L50 (-6.5, 69.8) -> (-14.5, 69.8)
  line L51 (-14.5, 69.8) -> (-14.5, 72.8)
  line L52 (-14.5, 62.8) -> (-6.5, 62.8) projected
  line L53 (-14.5, 62.8) -> (-6.5, 62.8)
  line L54 (-6.5, 62.8) -> (-6.5, 65.8)
  line L55 (-6.5, 65.8) -> (-14.5, 65.8)
  line L56 (-14.5, 65.8) -> (-14.5, 62.8)
  line L57 (-6.5, 42.8) -> (-14.5, 42.8) projected
  line L58 (-14.5, 42.8) -> (-6.5, 42.8)
  line L59 (-6.5, 42.8) -> (-6.5, 39.8)
  line L60 (-6.5, 39.8) -> (-14.5, 39.8)
  line L61 (-14.5, 39.8) -> (-14.5, 42.8)
  line L62 (-14.5, 32.8) -> (-6.5, 32.8)
  line L63 (-6.5, 32.8) -> (-6.5, 35.8)
  line L64 (-6.5, 35.8) -> (-14.5, 35.8)
  line L65 (-14.5, 35.8) -> (-14.5, 32.8)
  line L66 (-6.5, 12.8) -> (-14.5, 12.8) projected
  line L67 (-14.5, 12.8) -> (-6.5, 12.8)
  line L68 (-6.5, 12.8) -> (-6.5, 9.8)
  line L69 (-6.5, 9.8) -> (-14.5, 9.8)
  line L70 (-14.5, 9.8) -> (-14.5, 12.8)
  point P0 (0, 0)
  dimension "d404" = 8
  dimension "d405" = 3
  dimension "d406" = 8
  dimension "d407" = 3
  dimension "d408" = 8
  dimension "d409" = 3
  dimension "d410" = 8
  dimension "d411" = 3
  dimension "d412" = 8
  dimension "d413" = 3
  dimension "d414" = 3
  dimension "d415" = 8
  dimension "d416" = 3
  dimension "d417" = 8
  dimension "d418" = 3
  dimension "d419" = 8
  dimension "d420" = 3
  dimension "d421" = 8
  dimension "d422" = 3
  dimension "d423" = 8
  dimension "d424" = 3
  dimension "d425" = 8
  dimension "d426" = 3
  dimension "d427" = 8
  dimension "d428" = 3
  dimension "d429" = 8
  dimension "d430" = 3
  dimension "d431" = 8
  dimension "d432" = 3
  constraints: 120 end point, 30 parallel, 15 horizontal, 15 perpendicular, 3 point on line
  measures "d404" distance of L3.end L2.end
  measures "d405" distance of L2.end L1.end
  measures "d406" distance of L6.end L7.end
  measures "d407" distance of L5.end L6.end
  measures "d408" distance of L12.end L11.end
  measures "d409" distance of L11.end L10.end
  measures "d410" distance of L16.end L17.end
  measures "d411" distance of L15.end L16.end
  measures "d412" distance of L22.end L21.end
  measures "d413" distance of L21.end L20.end
  measures "d414" distance of L25.end L26.end
  measures "d415" distance of L31.end L30.end
  measures "d416" distance of L30.end L29.end
  measures "d417" distance of L35.end L36.end
  measures "d418" distance of L34.end L35.end
  measures "d419" distance of L41.end L40.end
  measures "d420" distance of L40.end L39.end
  measures "d421" distance of L46.end L45.end
  measures "d422" distance of L45.end L44.end
  measures "d423" distance of L49.end L50.end
  measures "d424" distance of L48.end L49.end
  measures "d425" distance of L55.end L54.end
  measures "d426" distance of L54.end L53.end
  measures "d427" distance of L59.end L60.end
  measures "d428" distance of L58.end L59.end
  measures "d429" distance of L64.end L63.end
  measures "d430" distance of L63.end L62.end
  measures "d431" distance of L68.end L69.end
  measures "d432" distance of L67.end L68.end
extrude "Extrusion47" add sketch "Sketch49" against normal blind 7 contours L4 L3 L2 L1 | L13 L12 L11 L9 | L15 L16 L17 L18 | L23 L22 L21 L19 | L26 L27 L28 L24 | L32 L31 L30 L29 | L34 L35 L36 L37 | L42 L41 L40 L39 | L47 L46 L45 L44 | L48 L49 L50 L51 | L56 L55 L54 L52 | L59 L60 L61 L57 | L65 L64 L63 L62 | L68 L69 L70 L66
sketch "Sketch50" plane through (0, 12, 0) normal (0, 1, 0) x (1, 0, 0)
  point P0 (0, 0)
sketch "Sketch51" plane through (0, 12, 0) normal (0, 1, 0) x (1, 0, 0)
  line L0 (-44.5, 102.8) -> (-36.5, 102.8)
  line L1 (-36.5, 102.8) -> (-36.5, 99.8)
  line L2 (-36.5, 99.8) -> (-44.5, 99.8)
  line L3 (-44.5, 99.8) -> (-44.5, 102.8)
  line L4 (-6.5, 102.8) -> (-14.5, 102.8) projected
  line L5 (-14.5, 102.8) -> (-6.5, 102.8)
  line L6 (-6.5, 102.8) -> (-6.5, 99.8)
  line L7 (-6.5, 99.8) -> (-14.5, 99.8)
  line L8 (-14.5, 99.8) -> (-14.5, 102.8)
  point P0 (0, 0)
  dimension "d435" = 8
  dimension "d436" = 3
  dimension "d437" = 8
  dimension "d438" = 3
  constraints: 16 end point, 4 parallel, 2 horizontal, 2 perpendicular
  measures "d435" distance of L1.end L2.end
  measures "d436" distance of L0.end L1.end
  measures "d437" distance of L6.end L7.end
  measures "d438" distance of L5.end L6.end
extrude "Extrusion48" add sketch "Sketch51" against normal blind 7
sketch "Sketch52" plane through (0, 12, 0) normal (0, 1, 0) x (1, 0, 0)
  line L0 (-44.5, 125.8) -> (-44.5, 99.8) projected
  line L1 (-44.5, 112.8) -> (-36.5, 112.8)
  line L2 (-36.5, 99.8) -> (-36.5, 125.8) projected
  line L3 (-14.5, 125.8) -> (-14.5, 99.8) projected
  line L4 (-14.5, 112.8) -> (-6.5, 112.8)
  line L5 (-6.5, 99.8) -> (-6.5, 125.8) projected
  line L6 (-6.5, 95.8) -> (-6.5, 69.8) projected
  line L7 (-6.5, 82.8) -> (-14.5, 82.8)
  line L8 (-36.5, 95.8) -> (-36.5, 69.8) projected
  line L9 (-36.5, 82.8) -> (-44.5, 82.8)
  line L10 (-44.5, 95.8) -> (-44.5, 69.8) projected
  line L11 (-44.5, 39.8) -> (-44.5, 65.8) projected
  line L12 (-44.5, 52.8) -> (-36.5, 52.8)
  line L13 (-36.5, 65.8) -> (-36.5, 39.8) projected
  line L14 (-14.5, 39.8) -> (-14.5, 65.8) projected
  line L15 (-14.5, 52.8) -> (-6.5, 52.8)
  line L16 (-6.5, 65.8) -> (-6.5, 39.8) projected
  line L17 (-6.5, 35.8) -> (-6.5, 9.8) projected
  line L18 (-6.5, 22.8) -> (-14.5, 22.8)
  line L19 (-14.5, 35.8) -> (-14.5, 9.8) projected
  line L20 (-36.5, 9.8) -> (-36.5, 35.8) projected
  line L21 (-36.5, 22.8) -> (-44.5, 22.8)
  line L22 (-44.5, 9.8) -> (-44.5, 35.8) projected
  line L23 (-40.5, 112.8) -> (-40.5, 124.3)
  line L24 (-40.5, 112.8) -> (-29, 112.8) construction
  line L25 (-40.5, 124.3) -> (-40.5, 101.3)
  line L26 (-10.5, 112.8) -> (-10.5, 124.3)
  line L27 (-10.5, 124.3) -> (-10.5, 101.3)
  line L28 (-10.5, 82.8) -> (-10.5, 94.3)
  line L29 (-10.5, 94.3) -> (-10.5, 71.3)
  line L30 (-40.5, 82.8) -> (-40.5, 94.3)
  line L31 (-40.5, 94.3) -> (-40.5, 71.3)
  line L32 (-40.5, 52.8) -> (-40.5, 64.3)
  line L33 (-40.5, 64.3) -> (-40.5, 41.3)
  line L34 (-40.5, 22.8) -> (-40.5, 34.3)
  line L35 (-40.5, 34.3) -> (-40.5, 11.3)
  line L36 (-10.5, 22.8) -> (-10.5, 34.3)
  line L37 (-10.5, 34.3) -> (-10.5, 11.3)
  line L38 (-10.5, 52.8) -> (-10.5, 64.3)
  line L39 (-10.5, 64.3) -> (-10.5, 41.3)
  line L40 (-40.5, 124.3) -> (-36.5, 120.3)
  line L41 (-40.5, 124.3) -> (-34.8431, 124.3) construction
  line L42 (-36.5, 120.3) -> (-40.5, 124.3)
  line L43 (-44.5, 120.3) -> (-40.5, 124.3)
  line L44 (-10.5, 124.3) -> (-14.5, 120.3)
  line L45 (-10.5, 124.3) -> (-6.5, 120.3)
  line L46 (-40.5, 101.3) -> (-44.5, 105.3)
  line L47 (-40.5, 101.3) -> (-36.5, 105.3)
  line L48 (-40.5, 94.3) -> (-36.5, 90.3)
  line L49 (-36.5, 90.3) -> (-40.5, 94.3)
  line L50 (-44.5, 90.3) -> (-40.5, 94.3)
  line L51 (-10.5, 94.3) -> (-14.5, 90.3)
  line L52 (-14.5, 90.3) -> (-10.5, 94.3)
  line L53 (-10.5, 94.3) -> (-6.5, 90.3)
  line L54 (-10.5, 71.3) -> (-6.5, 75.3)
  line L55 (-10.5, 71.3) -> (-14.5, 75.3)
  line L56 (-14.5, 69.8) -> (-14.5, 95.8) projected
  line L57 (-40.5, 71.3) -> (-36.5, 75.3)
  line L58 (-40.5, 71.3) -> (-44.5, 75.3)
  line L59 (-40.5, 64.3) -> (-36.5, 60.3)
  line L60 (-40.5, 64.3) -> (-44.5, 60.3)
  line L61 (-40.5, 41.3) -> (-36.5, 45.3)
  line L62 (-40.5, 41.3) -> (-44.5, 45.3)
  line L63 (-40.5, 34.3) -> (-36.5, 30.3)
  line L64 (-36.5, 30.3) -> (-40.5, 34.3)
  line L65 (-44.5, 30.3) -> (-40.5, 34.3)
  line L66 (-40.5, 11.3) -> (-44.5, 15.3)
  line L67 (-40.5, 11.3) -> (-36.5, 15.3)
  line L68 (-10.5, 34.3) -> (-6.5, 30.3)
  line L69 (-10.5, 34.3) -> (-14.5, 30.3)
  line L70 (-10.5, 11.3) -> (-6.5, 15.3)
  line L71 (-10.5, 11.3) -> (-14.5, 15.3)
  line L72 (-10.5, 64.3) -> (-14.5, 60.3)
  line L73 (-10.5, 64.3) -> (-6.5, 60.3)
  line L74 (-10.5, 41.3) -> (-6.5, 45.3)
  line L75 (-10.5, 41.3) -> (-14.5, 45.3)
  line L76 (-44.5, 125.8) -> (-36.5, 125.8)
  line L77 (-36.5, 125.8) -> (-36.5, 99.8)
  line L78 (-36.5, 99.8) -> (-44.5, 99.8)
  line L79 (-44.5, 99.8) -> (-44.5, 125.8)
  line L80 (-14.5, 125.8) -> (-6.5, 125.8)
  line L81 (-6.5, 125.8) -> (-6.5, 99.8)
  line L82 (-6.5, 99.8) -> (-14.5, 99.8)
  line L83 (-14.5, 99.8) -> (-14.5, 125.8)
  line L84 (-36.5, 69.8) -> (-44.5, 69.8) projected
  line L85 (-44.5, 95.8) -> (-36.5, 95.8)
  line L86 (-36.5, 95.8) -> (-36.5, 69.8)
  line L87 (-36.5, 69.8) -> (-44.5, 69.8)
  line L88 (-44.5, 69.8) -> (-44.5, 95.8)
  line L89 (-44.5, 65.8) -> (-36.5, 65.8)
  line L90 (-36.5, 65.8) -> (-36.5, 39.8)
  line L91 (-36.5, 39.8) -> (-44.5, 39.8)
  line L92 (-44.5, 39.8) -> (-44.5, 65.8)
  line L93 (-44.5, 35.8) -> (-36.5, 35.8) projected
  line L94 (-44.5, 35.8) -> (-36.5, 35.8)
  line L95 (-36.5, 35.8) -> (-36.5, 9.8)
  line L96 (-36.5, 9.8) -> (-44.5, 9.8)
  line L97 (-44.5, 9.8) -> (-44.5, 35.8)
  line L98 (-14.5, 35.8) -> (-6.5, 35.8) projected
  line L99 (-6.5, 35.8) -> (-14.5, 35.8)
  line L100 (-14.5, 35.8) -> (-14.5, 9.8)
  line L101 (-14.5, 9.8) -> (-6.5, 9.8)
  line L102 (-6.5, 9.8) -> (-6.5, 35.8)
  line L103 (-14.5, 65.8) -> (-6.5, 65.8) projected
  line L104 (-14.5, 65.8) -> (-6.5, 65.8)
  line L105 (-6.5, 65.8) -> (-6.5, 39.8)
  line L106 (-6.5, 39.8) -> (-14.5, 39.8)
  line L107 (-14.5, 39.8) -> (-14.5, 65.8)
  line L108 (-6.5, 69.8) -> (-14.5, 69.8) projected
  line L109 (-14.5, 95.8) -> (-6.5, 95.8)
  line L110 (-6.5, 95.8) -> (-6.5, 69.8)
  line L111 (-6.5, 69.8) -> (-14.5, 69.8)
  line L112 (-14.5, 69.8) -> (-14.5, 95.8)
  line L113 (-10.5, 101.3) -> (-6.5, 105.3)
  line L114 (-10.5, 101.3) -> (-14.5, 105.3)
  point P0 (0, 0)
  point P1 (-6.5, 9.8)
  dimension "d441" = 11.5
  dimension "d442" = 90
  dimension "d443" = 23
  dimension "d444" = 0
  dimension "d445" = 11.5
  dimension "d446" = 23
  dimension "d447" = 11.5
  dimension "d448" = 23
  dimension "d449" = 11.5
  dimension "d450" = 23
  dimension "d451" = 11.5
  dimension "d452" = 23
  dimension "d453" = 11.5
  dimension "d454" = 11.5
  dimension "d455" = 23
  dimension "d456" = 45
  constraints: 188 end point, 34 point on line, 27 perpendicular, 23 midpoint, 21 parallel, 11 horizontal, 8 vertical, 4 collinear, 2 equal length
  measures "d441" distance of L23.start L23.end
  measures "d442" angle of L24 L23
  measures "d443" distance of L23.end L25.end
  measures "d444" distance between parallel lines of L25 L23
  measures "d445" distance of L26.start L26.end
  measures "d446" distance of L26.end L27.end
  measures "d447" distance of L28.start L28.end
  measures "d448" distance of L28.end L29.end
  measures "d449" distance of L32.start L32.end
  measures "d450" distance of L32.end L33.end
  measures "d451" distance of L34.start L34.end
  measures "d452" distance of L34.end L35.end
  measures "d453" distance of L36.start L36.end
  measures "d454" distance of L38.start L38.end
  measures "d455" distance of L38.end L39.end
  measures "d456" angle of L40 L41
extrude "Extrusion49" add sketch "Sketch52" along normal blind 4 contours L76 L2 L40 L43 L0 | L46 L47 L2 L78 L0 | L80 L5 L45 L44 L3 | L114 L113 L5 L82 L3 | L6 L53 L51 L56 L109 | L6 L108 L56 L55 L54 | L8 L48 L50 L10 L85 | L8 L84 L10 L58 L57 | L11 L62 L61 L13 L91 | L11 L89 L13 L59 L60 | L14 L75 L74 L16 L106 | L14 L103 L16 L73 L72 | L17 L68 L69 L19 L98 | L17 L101 L19 L71 L70 | L96 L22 L66 L67 L20 | L63 L65 L22 L93 L20
chamfer "Chamfer57" distance 2 distance2 3 2 edges at (-42.5, 16, -122.3) (-38.5, 16, -122.3)
chamfer "Chamfer58" distance 2 distance2 3 2 edges at (-42.5, 16, -103.3) (-38.5, 16, -103.3)
chamfer "Chamfer59" distance 2 distance2 3 2 edges at (-42.5, 16, -92.3) (-38.5, 16, -92.3)
chamfer "Chamfer60" distance 2 distance2 3 2 edges at (-42.5, 16, -73.3) (-38.5, 16, -73.3)
chamfer "Chamfer61" distance 2 distance2 3 2 edges at (-38.5, 16, -62.3) (-42.5, 16, -62.3)
chamfer "Chamfer62" distance 2 distance2 3 2 edges at (-42.5, 16, -43.3) (-38.5, 16, -43.3)
chamfer "Chamfer63" distance 2 distance2 3 2 edges at (-42.5, 16, -13.3) (-38.5, 16, -13.3)
chamfer "Chamfer64" distance 2 distance2 3 2 edges at (-42.5, 16, -32.3) (-38.5, 16, -32.3)
chamfer "Chamfer65" distance 2 distance2 3 2 edges at (-8.5, 16, -122.3) (-12.5, 16, -122.3)
chamfer "Chamfer66" distance 2 distance2 3 2 edges at (-12.5, 16, -103.3) (-8.5, 16, -103.3)
chamfer "Chamfer67" distance 2 distance2 3 2 edges at (-8.5, 16, -92.3) (-12.5, 16, -92.3)
chamfer "Chamfer68" distance 2 distance2 3 2 edges at (-12.5, 16, -73.3) (-8.5, 16, -73.3)
chamfer "Chamfer69" distance 2 distance2 3 1 edges at (-12.5, 16, -62.3) measured on face at (-12.8536, 16, -62.6536)
chamfer "Chamfer70" distance 2 distance2 3 2 edges at (-11.2071, 16, -65.0071) (-8.5, 16, -62.3)
chamfer "Chamfer71" distance 2 distance2 3 2 edges at (-12.5, 16, -43.3) (-8.5, 16, -43.3)
chamfer "Chamfer72" distance 2 distance2 3 2 edges at (-12.5, 16, -32.3) (-8.5, 16, -32.3)
chamfer "Chamfer73" distance 2 distance2 3 2 edges at (-12.5, 16, -13.3) (-8.5, 16, -13.3)
sketch "Sketch53" plane through (0, 12, 0) normal (0, 1, 0) x (1, 0, 0)
  line L0 (-70.5, 101.3) -> (-66.5, 105.3) projected
  line L1 (-66.5, 105.3) -> (-66.5, 120.3) projected
  line L2 (-66.5, 120.3) -> (-70.5, 124.3) projected
  line L3 (-70.5, 124.3) -> (-74.5, 120.3) projected
  line L4 (-74.5, 120.3) -> (-74.5, 105.3) projected
  line L5 (-74.5, 105.3) -> (-70.5, 101.3) projected
  line L6 (-40.5, 101.3) -> (-36.5, 105.3) projected
  line L7 (-36.5, 105.3) -> (-36.5, 120.3) projected
  line L8 (-36.5, 120.3) -> (-40.5, 124.3) projected
  line L9 (-40.5, 124.3) -> (-44.5, 120.3) projected
  line L10 (-44.5, 120.3) -> (-44.5, 105.3) projected
  line L11 (-44.5, 105.3) -> (-40.5, 101.3) projected
  line L12 (-10.5, 124.3) -> (-14.5, 120.3) projected
  line L13 (-14.5, 120.3) -> (-14.5, 105.3) projected
  line L14 (-14.5, 105.3) -> (-10.5, 101.3) projected
  line L15 (-10.5, 101.3) -> (-6.5, 105.3) projected
  line L16 (-6.5, 105.3) -> (-6.5, 120.3) projected
  line L17 (-6.5, 120.3) -> (-10.5, 124.3) projected
  line L18 (-6.5, 75.3) -> (-6.5, 90.3) projected
  line L19 (-10.5, 71.3) -> (-6.5, 75.3) projected
  line L20 (-6.5, 75.3) -> (-6.5, 90.3) projected
  line L21 (-6.5, 90.3) -> (-10.5, 94.3) projected
  line L22 (-10.5, 94.3) -> (-14.5, 90.3) projected
  line L23 (-14.5, 90.3) -> (-14.5, 75.3) projected
  line L24 (-14.5, 75.3) -> (-10.5, 71.3) projected
  line L25 (-40.5, 71.3) -> (-36.5, 75.3) projected
  line L26 (-36.5, 75.3) -> (-36.5, 90.3) projected
  line L27 (-36.5, 90.3) -> (-40.5, 94.3) projected
  line L28 (-40.5, 94.3) -> (-44.5, 90.3) projected
  line L29 (-44.5, 90.3) -> (-44.5, 75.3) projected
  line L30 (-44.5, 75.3) -> (-40.5, 71.3) projected
  line L31 (-70.5, 71.3) -> (-66.5, 75.3) projected
  line L32 (-66.5, 75.3) -> (-66.5, 90.3) projected
  line L33 (-66.5, 90.3) -> (-70.5, 94.3) projected
  line L34 (-70.5, 94.3) -> (-74.5, 90.3) projected
  line L35 (-74.5, 90.3) -> (-74.5, 75.3) projected
  line L36 (-74.5, 75.3) -> (-70.5, 71.3) projected
  line L37 (-70.5, 64.3) -> (-74.5, 60.3) projected
  line L38 (-74.5, 60.3) -> (-74.5, 45.3) projected
  line L39 (-74.5, 45.3) -> (-70.5, 41.3) projected
  line L40 (-70.5, 41.3) -> (-66.5, 45.3) projected
  line L41 (-66.5, 45.3) -> (-66.5, 60.3) projected
  line L42 (-66.5, 60.3) -> (-70.5, 64.3) projected
  line L43 (-40.5, 41.3) -> (-36.5, 45.3) projected
  line L44 (-36.5, 45.3) -> (-36.5, 60.3) projected
  line L45 (-36.5, 60.3) -> (-40.5, 64.3) projected
  line L46 (-40.5, 64.3) -> (-44.5, 60.3) projected
  line L47 (-44.5, 60.3) -> (-44.5, 45.3) projected
  line L48 (-44.5, 45.3) -> (-40.5, 41.3) projected
  line L49 (-10.5, 64.3) -> (-14.5, 60.3) projected
  line L50 (-14.5, 60.3) -> (-14.5, 45.3) projected
  line L51 (-14.5, 45.3) -> (-10.5, 41.3) projected
  line L52 (-10.5, 41.3) -> (-6.5, 45.3) projected
  line L53 (-6.5, 45.3) -> (-6.5, 60.3) projected
  line L54 (-6.5, 60.3) -> (-10.5, 64.3) projected
  line L55 (-10.5, 11.3) -> (-6.5, 15.3) projected
  line L56 (-6.5, 15.3) -> (-6.5, 30.3) projected
  line L57 (-6.5, 30.3) -> (-10.5, 34.3) projected
  line L58 (-10.5, 34.3) -> (-14.5, 30.3) projected
  line L59 (-14.5, 30.3) -> (-14.5, 15.3) projected
  line L60 (-14.5, 15.3) -> (-10.5, 11.3) projected
  line L61 (-40.5, 11.3) -> (-36.5, 15.3) projected
  line L62 (-36.5, 15.3) -> (-36.5, 30.3) projected
  line L63 (-36.5, 30.3) -> (-40.5, 34.3) projected
  line L64 (-40.5, 34.3) -> (-44.5, 30.3) projected
  line L65 (-44.5, 30.3) -> (-44.5, 15.3) projected
  line L66 (-44.5, 15.3) -> (-40.5, 11.3) projected
  line L67 (-66.5, 15.3) -> (-66.5, 30.3) projected
  line L68 (-70.5, 11.3) -> (-66.5, 15.3) projected
  line L69 (-66.5, 15.3) -> (-66.5, 30.3) projected
  line L70 (-66.5, 30.3) -> (-70.5, 34.3) projected
  line L71 (-70.5, 34.3) -> (-74.5, 30.3) projected
  line L72 (-74.5, 30.3) -> (-74.5, 15.3) projected
  line L73 (-74.5, 15.3) -> (-70.5, 11.3) projected
  point P0 (0, 0)
extrude "Extrusion50" cut sketch "Sketch53" against normal blind 2
sketch "Sketch54" plane through (0, 10, 0) normal (0, 1, 0) x (1, 0, 0)
  line L0 (-83.25, 131.7) -> (2.25, 131.7) projected
  line L1 (2.25, 3.9) -> (2.25, 131.7) projected
  line L2 (-83.25, 131.7) -> (2.25, 131.7)
  line L3 (2.25, 131.7) -> (2.25, 3.9)
  line L4 (2.25, 3.9) -> (-83.25, 3.9)
  line L5 (-83.25, 3.9) -> (-83.25, 131.7)
  point P0 (0, 0)
  constraints: 8 end point, 2 parallel, 1 horizontal, 1 perpendicular
extrude "Extrusion51" cut sketch "Sketch54" along normal blind 10
sketch "Sketch55" plane through (0, 5, 0) normal (0, 1, 0) x (1, 0, 0)
  line L0 (-74.5, 125.8) -> (-66.5, 125.8) projected
  line L1 (-66.5, 35.8) -> (-66.5, 9.8) projected
  line L2 (-74.5, 125.8) -> (-66.5, 125.8)
  line L3 (-66.5, 125.8) -> (-66.5, 9.8)
  line L4 (-66.5, 9.8) -> (-74.5, 9.8)
  line L5 (-74.5, 9.8) -> (-74.5, 125.8)
  line L6 (-44.5, 125.8) -> (-36.5, 125.8) projected
  line L7 (-36.5, 9.8) -> (-44.5, 9.8) projected
  line L8 (-44.5, 125.8) -> (-36.5, 125.8)
  line L9 (-36.5, 125.8) -> (-36.5, 9.8)
  line L10 (-36.5, 9.8) -> (-44.5, 9.8)
  line L11 (-44.5, 9.8) -> (-44.5, 125.8)
  line L12 (-14.5, 125.8) -> (-6.5, 125.8) projected
  line L13 (-14.5, 125.8) -> (-6.5, 125.8)
  line L14 (-6.5, 125.8) -> (-6.5, 9.8)
  line L15 (-6.5, 9.8) -> (-14.5, 9.8)
  line L16 (-14.5, 9.8) -> (-14.5, 125.8)
  point P0 (0, 0)
  constraints: 24 end point, 6 parallel, 3 horizontal, 3 perpendicular, 1 point on line
extrude "Extrusion52" add sketch "Sketch55" along normal blind 5
sketch "Sketch56" plane through (0, 10, 0) normal (0, 1, 0) x (1, 0, 0)
  point P0 (0, 0)